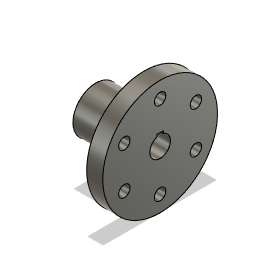
Half-coupling1 (Autodesk Fusion 360 design; units mm, degrees)
Autodesk Fusion 360 part; units mm, degrees
note: some values were not read from the file. Chosen so that the rebuilt part matches the saved one: which face or edge a step refers to.
sketch "Sketch1" plane through (0, 0, 0) normal (0, 0, 1) x (1, 0, 0)
  line L0 (-70, 0) -> (70, 0)
  line L1 (-70, 0) -> (-70, 50)
  line L2 (70, 125) -> (70, 0)
  line L3 (35, 125) -> (70, 125)
  line L4 (-70, 50) -> (35, 50)
  line L5 (35, 125) -> (35, 50)
revolve "Revolve1" add sketch "Sketch1" angle 360 about axis through (-70, 0, 0) along (1, 0, 0)
sketch "Sketch2" plane through (0, 0, 0) normal (1, 0, 0) x (0, 0, -1)
  arc A0 (-7, 21.383) -> (7, 21.383) centre (0, -0.0002) ccw
  line L0 (-6.75, 26.3) -> (6.75, 26.3)
  line L1 (-7, 26.05) -> (-7, 21.383)
  line L2 (7, 26.05) -> (7, 21.383)
  arc A1 (-6.75, 26.3) -> (-7, 26.05) centre (-6.75, 26.05) ccw
  arc A2 (7, 26.05) -> (6.75, 26.3) centre (6.75, 26.05) ccw
  constraint tangent L0 A1
  constraint tangent L1 A1
  constraint tangent L2 A2
  constraint tangent L0 A2
extrude "Extrude1" cut sketch "Sketch2" along normal mid plane 140
sketch "Sketch3" plane through (0, 0, 0) normal (1, 0, 0) x (0, 0, -1)
  circle A0 through (9, 90, 35) (-4.5, 97.7942, 35) (-4.5, 82.2058, 35)
sketch "Sketch4" plane through (0, 0, 0) normal (1, 0, 0) x (0, 0, -1)
  circle A0 through (12.5, 90, 70) (-6.25, 100.8253, 70) (-6.25, 79.1747, 70)
sketch "Sketch3 (curves 35 mm off its plane)" plane through (35, 0, 0) normal (1, 0, 0) x (0, 0, -1)
  circle A0 centre (0, 90) radius 9
sketch "Sketch4 (curves 70 mm off its plane)" plane through (70, 0, 0) normal (1, 0, 0) x (0, 0, -1)
  circle A0 centre (0, 90) radius 12.5
loft "Loft1" cut profiles "Sketch3 (curves 35 mm off its plane)", "Sketch4 (curves 70 mm off its plane)" section 1 section 2
pattern_circular "C-Pattern1" count 6 over 360 about axis through (1.75, 0, 0) along (1, 0, 0) of 1 faces at (66.1111, 91.8051, -11.9758)
equation "angle = 360.0 deg"
equation "symmetricDistance = 70.00 mm"
equation "taperAngle1 = 0.0 deg"
equation "countU = 6"
equation "TotalAngle = 360 deg"
